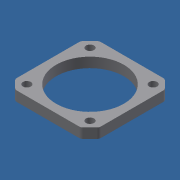
# Autodesk Inventor part: StepperXYHolder
Saved by Autodesk Inventor 2018 (Build 220112000, 112)
## iProperties
Created: 2022-08-30
Part Number: StepperXYHolder
Material: Generic
Document SubType Name: Modeling
Designer: Nathann
Density: 1 g/cm^3
Appearance: Default
Author: Nathann
Autodesk Inventor part; units mm, degrees
ref_plane "YZ Plane" through (0, 0, 0) normal (1, 0, 0) x (0, 1, 0)
ref_plane "XZ Plane" through (0, 0, 0) normal (0, 1, 0) x (-1, 0, 0)
ref_plane "XY Plane" through (0, 0, 0) normal (0, 0, 1) x (1, 0, 0)
sketch "Sketch1" plane through (0, 0, 0) normal (0, 0, 1) x (1, 0, 0)
  arc A0 (-20.5392, 17.1146) -> (-21.125, 15.7004) centre (-19.125, 15.7004) ccw projected
  line L0 (-21.125, -15.7004) -> (-21.125, 15.7004) projected
  arc A1 (-21.125, -15.7004) -> (-20.5392, -17.1146) centre (-19.125, -15.7004) ccw projected
  line L1 (-20.5392, -17.1146) -> (-17.1146, -20.5392) projected
  arc A2 (-17.1146, -20.5392) -> (-15.7004, -21.125) centre (-15.7004, -19.125) ccw projected
  line L2 (15.7004, -21.125) -> (-15.7004, -21.125) projected
  arc A3 (15.7004, -21.125) -> (17.1146, -20.5392) centre (15.7004, -19.125) ccw projected
  line L3 (20.5392, -17.1146) -> (17.1146, -20.5392) projected
  arc A4 (20.5392, -17.1146) -> (21.125, -15.7004) centre (19.125, -15.7004) ccw projected
  line L4 (21.125, 15.7004) -> (21.125, -15.7004) projected
  arc A5 (21.125, 15.7004) -> (20.5392, 17.1146) centre (19.125, 15.7004) ccw projected
  line L5 (20.5392, 17.1146) -> (17.1146, 20.5392) projected
  arc A6 (17.1146, 20.5392) -> (15.7004, 21.125) centre (15.7004, 19.125) ccw projected
  line L6 (-15.7004, 21.125) -> (15.7004, 21.125) projected
  arc A7 (-15.7004, 21.125) -> (-17.1146, 20.5392) centre (-15.7004, 19.125) ccw projected
  line L7 (-20.5392, 17.1146) -> (-17.1146, 20.5392) projected
  circle A8 centre (0, 0) radius 16 projected
  circle A9 centre (-15.875, -15.875) radius 1.625 projected
  circle A10 centre (15.875, 15.875) radius 1.625 projected
  circle A11 centre (-15.875, 15.875) radius 1.625 projected
  circle A12 centre (15.875, -15.875) radius 1.625 projected
  circle A13 centre (0, 0) radius 12
  circle A14 centre (-15.875, 15.875) radius 2
  circle A15 centre (15.875, 15.875) radius 2
  circle A16 centre (15.875, -15.875) radius 2
  circle A17 centre (-15.875, -15.875) radius 2
  point P0 (0, 0)
  dimension "d0" = 24
  dimension "d1" = 4
  dimension "d2" = 4
  dimension "d3" = 4
  dimension "d4" = 4
  constraints: 5 centre point, 4 coincident
  measures "d0" diameter of A13
  measures "d1" diameter of A14
  measures "d2" diameter of A15
  measures "d3" diameter of A16
  measures "d4" diameter of A17
extrude "Extrusion1" add sketch "Sketch1" along normal blind 5 contours L7 A7 L6 A6 L5 A5 L4 A4 L3 A3 L2 A2 L1 A1 L0 A0 | A8
sketch "Sketch3" plane through (0, 0, 5) normal (0, 0, 1) x (1, 0, 0)
  line L0 (-15.7004, 21.125) -> (15.7004, 21.125) projected
  line L1 (15.7004, 21.125) -> (-46.125, 21.125)
  line L2 (-46.125, 21.125) -> (-46.125, 26.125)
  line L3 (-46.125, 26.125) -> (15.7004, 26.125)
  line L4 (15.7004, 26.125) -> (15.7004, 21.125)
  line L5 (-21.125, 15.7004) -> (-21.125, -15.7004) projected
  line L6 (-21.125, -15.7004) -> (-26.125, -15.7004)
  line L7 (-26.125, -15.7004) -> (-26.125, 46.125)
  line L8 (-26.125, 46.125) -> (-21.125, 46.125)
  line L9 (-21.125, 46.125) -> (-21.125, -15.7004)
  point P0 (0, 0)
  dimension "d11" = 5
  dimension "d12" = 5
  dimension "d13" = 20
  dimension "d14" = 20
  constraints: 16 end point, 4 parallel, 2 horizontal, 2 perpendicular
  measures "d11" distance of L7.end L8.end
  measures "d12" distance of L1.end L2.end
  measures "d13" distance between parallel lines of L2 L7
  measures "d14" distance between parallel lines of L8 L3
extrude "Extrusion3" add sketch "Sketch3" against normal blind 40
sketch "Sketch4" plane through (0, 0, 5) normal (0, 0, 1) x (1, 0, 0)
  arc A0 (-15.7004, 21.125) -> (-17.1146, 20.5392) centre (-15.7004, 19.125) ccw projected
  line L0 (-17.1146, 20.5392) -> (-20.5392, 17.1146) projected
  arc A1 (-20.5392, 17.1146) -> (-21.125, 15.7004) centre (-19.125, 15.7004) ccw projected
  line L1 (-21.125, 21.125) -> (-21.125, 15.7004) projected
  line L2 (-15.7004, 21.125) -> (-21.125, 21.125) projected
  circle A2 centre (0, 0) radius 12 projected
  circle A3 centre (-15.875, -15.875) radius 2 projected
  circle A4 centre (15.875, -15.875) radius 2 projected
  circle A5 centre (15.875, 15.875) radius 2 projected
  circle A6 centre (-15.875, 15.875) radius 2 projected
  line L3 (15.7004, 26.125) -> (15.7004, 21.125) projected
  line L4 (-21.125, 26.125) -> (15.7004, 26.125) projected
  line L5 (-21.125, 46.125) -> (-21.125, 26.125) projected
  line L6 (-26.125, 46.125) -> (-21.125, 46.125) projected
  line L7 (-26.125, 26.125) -> (-26.125, 46.125) projected
  line L8 (-46.125, 26.125) -> (-26.125, 26.125) projected
  line L9 (-46.125, 21.125) -> (-46.125, 26.125) projected
  line L10 (-26.125, 21.125) -> (-46.125, 21.125) projected
  line L11 (-26.125, -15.7004) -> (-26.125, 21.125) projected
  line L12 (-21.125, -15.7004) -> (-26.125, -15.7004) projected
  arc A7 (-21.125, -15.7004) -> (-20.5392, -17.1146) centre (-19.125, -15.7004) ccw projected
  line L13 (-20.5392, -17.1146) -> (-17.1146, -20.5392) projected
  arc A8 (-17.1146, -20.5392) -> (-15.7004, -21.125) centre (-15.7004, -19.125) ccw projected
  line L14 (-15.7004, -21.125) -> (15.7004, -21.125) projected
  arc A9 (15.7004, -21.125) -> (17.1146, -20.5392) centre (15.7004, -19.125) ccw projected
  line L15 (17.1146, -20.5392) -> (20.5392, -17.1146) projected
  arc A10 (20.5392, -17.1146) -> (21.125, -15.7004) centre (19.125, -15.7004) ccw projected
  line L16 (21.125, -15.7004) -> (21.125, 15.7004) projected
  arc A11 (21.125, 15.7004) -> (20.5392, 17.1146) centre (19.125, 15.7004) ccw projected
  line L17 (20.5392, 17.1146) -> (17.1146, 20.5392) projected
  arc A12 (17.1146, 20.5392) -> (15.7004, 21.125) centre (15.7004, 19.125) ccw projected
  point P0 (0, 0)
extrude "Extrusion4" add sketch "Sketch4" against normal blind 5 contours A0 L0 A1 L1 L2
sketch "Sketch5" plane through (-21.125, 26.125, 5) normal (1, 0, 0) x (0, 0, -1)
  circle A0 centre (10, 10) radius 2.5
  circle A1 centre (30, 10) radius 2.5
  line L0 (0, 20) -> (40, 20) projected
  line L1 (0, 20) -> (0, 0) projected
  point P0 (5, -26.125)
  dimension "d19" = 5
  dimension "d20" = 5
  dimension "d21" = 10
  dimension "d22" = 10
  dimension "d23" = 20
  dimension "d24" = 10
  constraints: 2 centre point
  measures "d19" diameter of A0
  measures "d20" diameter of A1
  measures "d21" distance from line of A0.centre L0
  measures "d22" distance from line of L0 A1.centre
  measures "d23" distance of A1.centre A0.centre
  measures "d24" distance from line of L1 A0.centre
extrude "Extrusion5" cut sketch "Sketch5" against normal through all
sketch "Sketch6" plane through (-46.125, 21.125, 5) normal (0, -1, 0) x (1, 0, 0)
  circle A0 centre (10, -30) radius 2.5
  circle A1 centre (10, -10) radius 2.5
  line L0 (0, 0) -> (0, -40) projected
  line L1 (20, 0) -> (0, 0) projected
  point P0 (46.125, -5)
  dimension "d27" = 10
  dimension "d28" = 10
  dimension "d29" = 5
  dimension "d30" = 5
  dimension "d31" = 20
  dimension "d32" = 10
  constraints: 2 centre point
  measures "d27" distance from line of L0 A0.centre
  measures "d28" distance from line of L0 A1.centre
  measures "d29" diameter of A1
  measures "d30" diameter of A0
  measures "d31" distance of A0.centre A1.centre
  measures "d32" distance from line of L1 A1.centre
extrude "Extrusion6" cut sketch "Sketch6" against normal through all
sketch "Sketch7" plane through (0, 0, -35) normal (0, 0, -1) x (-1, 0, 0)
  line L0 (21.625, 21.625) -> (-23.2924, 21.625)
  line L1 (-23.2924, 21.625) -> (-23.2924, -21.9013)
  line L2 (-23.2924, -21.9013) -> (21.625, -21.9013)
  line L3 (21.625, -21.9013) -> (21.625, 21.625)
  line L4 (-15.7004, 21.125) -> (21.125, 21.125) projected
  line L5 (21.125, 21.125) -> (21.125, -15.7004) projected
  point P0 (0, 0)
  dimension "d35" = 0.5
  dimension "d36" = 0.5
  constraints: 8 end point, 2 parallel, 1 horizontal, 1 perpendicular
  measures "d35" distance between parallel lines of L4 L0
  measures "d36" distance between parallel lines of L3 L5
extrude "Extrusion7" cut sketch "Sketch7" against normal blind 35
equation "\"d36\" = d35"
body "Solid1"
